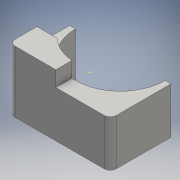
# Autodesk Inventor part: 240503_3Dsketch12
Saved by Autodesk Inventor 2016 (Build 200138000, 138)
## iProperties
Created: 2024-05-03
Part Number: 240503_3Dsketch12
Material: 일반
Document SubType Name: Modeling
Designer: pc
Density: 1 g/cm^3
Appearance: 기본값
Author: pc
Autodesk Inventor part; units mm, degrees
ref_plane "YZ Plane" through (0, 0, 0) normal (1, 0, 0) x (0, 1, 0)
ref_plane "XZ Plane" through (0, 0, 0) normal (0, 1, 0) x (-1, 0, 0)
ref_plane "XY Plane" through (0, 0, 0) normal (0, 0, 1) x (1, 0, 0)
sketch "스케치1" plane through (0, 0, 0) normal (0, 0, 1) x (1, 0, 0)
  line L0 (16.3992, -9.8355) -> (-16.3992, -9.8355)
  line L1 (-16.3992, -9.8355) -> (-16.3992, 9.8355)
  line L2 (-16.3992, 9.8355) -> (16.3992, 9.8355)
  line L3 (16.3992, 9.8355) -> (16.3992, -9.8355)
  line L4 (16.3992, -9.8355) -> (-16.3992, 9.8355) construction
  line L5 (-16.3992, -9.8355) -> (16.3992, 9.8355) construction
  point P0 (0, 0)
  constraints: 12 end point, 2 midpoint, 2 parallel, 1 horizontal, 1 perpendicular
extrude "돌출1" add sketch "스케치1" along normal blind 15
sketch "스케치2" plane through (0, 0, 15) normal (0, 0, 1) x (1, 0, 0)
  line L0 (-16.3992, 9.8355) -> (-16.3992, -9.8355) projected
  line L1 (-16.3992, -9.8355) -> (16.3992, -9.8355) projected
  line L2 (-16.3992, -0.8122) -> (-1.2307, -0.8122)
  line L3 (-1.2307, -0.8122) -> (-1.2307, -9.8355)
  line L4 (-1.2307, -9.8355) -> (-16.3992, -9.8355)
  line L5 (-16.3992, -9.8355) -> (-16.3992, -0.8122)
  point P0 (0, 0)
  constraints: 8 end point, 2 parallel, 2 point on line, 1 horizontal, 1 perpendicular
extrude "돌출2" add sketch "스케치2" along normal blind 5
sketch "스케치3" plane through (0, 0, 15) normal (0, 0, 1) x (1, 0, 0)
  point P0 (0, 0)
sketch "스케치4" plane through (0, 0, 0) normal (0, 0, -1) x (-1, 0, 0)
  line L0 (-16.3992, 9.8355) -> (16.3992, 9.8355) projected
  circle A0 centre (0, 9.8355) radius 14.5299
  point P0 (0, 0)
  constraints: 1 centre point, 1 midpoint
extrude "돌출3" cut sketch "스케치4" against normal blind 20
fillet "모깎기1" radius 2 1 edges at (16.3992, -9.8355, 7.5)
fillet "모깎기2" radius 2 1 edges at (-16.3992, -9.8355, 10)
